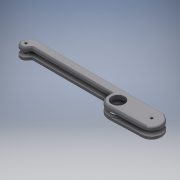
# Autodesk Inventor part: Arm 20X - forearm r
Saved by Autodesk Inventor 2017 (Build 210142000, 142)
## iProperties
Created: 2016-03-29
Part Number: Arm 20X - forearm r
Material: Generic
Document SubType Name: Modeling
Designer: Ali
Density: 1 g/cm^3
Appearance: Default
Author: Ali
Autodesk Inventor part; units mm, degrees
ref_plane "YZ Plane" through (0, 0, 0) normal (1, 0, 0) x (0, 1, 0)
ref_plane "XZ Plane" through (0, 0, 0) normal (0, 1, 0) x (-1, 0, 0)
sketch "Sketch1" plane through (0, 0, 0) normal (0, 0, 1) x (1, 0, 0)
  circle A0 centre (0, 0) radius 11
  circle A1 centre (-160, 5.5) radius 2.15
  circle A2 centre (54.4, 2) radius 2.15
  arc A3 (54.9829, -15.1401) -> (63.0119, 16.831) centre (54.4, 2) ccw
  arc A4 (-166.8053, 11) -> (-153.1947, 0) centre (-160, 5.5) ccw
  arc A5 (-17, 0) -> (0.5778, -16.9902) centre (0, 0) ccw
  line L0 (-262.8088, 0) -> (191.982, 0) construction
  line L1 (54.9829, -15.1401) -> (0.5778, -16.9902)
  line L2 (63.0119, 16.831) -> (57.1634, 20.227)
  line L3 (57.1634, 20.227) -> (-159.3481, 20.227)
  line L4 (-159.3481, 20.227) -> (-166.8053, 11)
  line L5 (-17, 0) -> (-17, 5.239)
  line L6 (-17, 5.239) -> (-148.9605, 5.239)
  line L7 (-148.9605, 5.239) -> (-153.1947, 0)
  dimension "d0" = 22
  dimension "d1" = 4.3
  dimension "d2" = 160
  dimension "d3" = 5.5
  dimension "d4" = 4.3
  dimension "d5" = 54.4
  dimension "d6" = 2
  dimension "d7" = 15
  dimension "d9" = 6
  dimension "d20" = 6.6
  constraints: 16 end point, 7 point on circle, 6 centre point, 6 tangent, 3 horizontal, 3 point on line, 1 coincident, 1 parallel, 1 vertical
  measures "d0" diameter of A0
  measures "d1" diameter of A1
  measures "d2" horizontal distance of A1.centre point (0, 0)
  measures "d3" vertical distance of A1.centre point (0, 0)
  measures "d4" diameter of A2
  measures "d5" horizontal distance of A2.centre point (0, 0)
  measures "d6" vertical distance of A2.centre point (0, 0)
  measures "d7" radial gap between concentric circles of A2 A3
  measures "d9" radial gap between concentric circles of A0 A5
  measures "d20" radial gap between concentric circles of A4 A1
extrude "Extrusion1" add sketch "Sketch1" along normal blind 6
sketch "Sketch2" plane through (0, 0, 6) normal (0, 0, 1) x (1, 0, 0)
  circle A0 centre (0, 0) radius 11 projected
  circle A1 centre (0, 0) radius 17
  constraints: 1 centre point, 1 coincident
extrude "Extrusion2" add sketch "Sketch2" along normal blind 1
fillet "Fillet2" radius 3 5 edges at (-165.5, -1.3053, 0) (-11.8148, -12.2234, 0) (71.0335, -2.1772, 0) (-51.0924, 20.227, 0) (-82.9803, 5.239, 0)
ref_plane "Work Plane1" through (0, 0, 10.3) normal (0, 0, -1) x (-1, 0, 0)
mirror "Mirror2" about plane through (0, 0, 10.3) normal (0, 0, -1) of "Extrusion1", "Fillet2", "Extrusion2"
body "Solid1"
